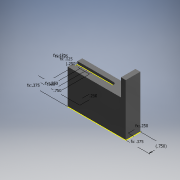
# Autodesk Inventor part: Spring block
Saved by Autodesk Inventor 2019 (Build 230136000, 136)
## iProperties
Part Number: Spring block
Material: Generic
Document SubType Name: Modeling
Designer: Delta
Appearance: Default
Author: Delta
Autodesk Inventor part; units mm, degrees
ref_plane "YZ Plane" through (0, 0, 0) normal (1, 0, 0) x (0, 1, 0)
ref_plane "XZ Plane" through (0, 0, 0) normal (0, 1, 0) x (-1, 0, 0)
ref_plane "XY Plane" through (0, 0, 0) normal (0, 0, 1) x (1, 0, 0)
sketch "Sketch1" plane through (0, 0, 0) normal (0, 0, 1) x (1, 0, 0)
  line L0 (0, 0) -> (76.2, 0)
  line L1 (76.2, 0) -> (76.2, 68.2498)
  line L2 (76.2, 68.2498) -> (0, 68.2498)
  line L3 (0, 68.2498) -> (0, 0)
  line L4 (0, 68.2498) -> (69.85, 68.2498)
  line L5 (69.85, 68.2498) -> (69.85, 45.3898)
  line L6 (69.85, 45.3898) -> (0, 45.3898)
  line L7 (0, 45.3898) -> (0, 68.2498)
  dimension "d0" = 76.2
  dimension "d1" = 68.2498
  dimension "d2" = 69.85
  dimension "d3" = 22.86
  constraints: 16 end point, 4 parallel, 2 horizontal, 2 perpendicular
  measures "d0" distance of L2.end L1.end
  measures "d1" distance of L1.end L0.end
  measures "d2" distance of L5.end L6.end
  measures "d3" distance of L4.end L5.end
extrude "Extrusion1" add sketch "Sketch1" along normal blind 19.05 contours L3 L6 L5 L2 L1 L0
sketch "Sketch2" plane through (0, 45.3898, 0) normal (0, 1, 0) x (1, 0, 0)
  line L0 (0, 0) -> (0, -19.05) projected
  line L1 (0, -6.35) -> (47.625, -6.35)
  line L2 (47.625, -6.35) -> (47.625, -12.7)
  line L3 (47.625, -12.7) -> (0, -12.7)
  line L4 (0, -12.7) -> (0, -6.35)
  line L5 (0, 0) -> (69.85, 0) projected
  circle A0 centre (47.625, -9.525) radius 3.175
  dimension "d6" = 47.625
  dimension "d7" = 6.35
  dimension "d8" = 6.35
  constraints: 8 end point, 2 parallel, 1 horizontal, 1 midpoint, 1 perpendicular, 1 point on line, 1 vertical alignment, 2 other
  measures "d6" distance of L2.end L3.end
  measures "d7" distance between parallel lines of L3 L1
  measures "d8" distance between parallel lines of L5 L1
extrude "Extrusion2" cut sketch "Sketch2" against normal blind 3.7084
sketch "Sketch3" plane through (0, 41.6814, 0) normal (0, 1, 0) x (1, 0, 0)
  line L0 (47.625, -12.7) -> (0, -12.7) projected
  line L1 (0, -6.35) -> (47.625, -6.35) projected
  line L2 (0, -12.7) -> (0, -6.35) projected
  point P0 (0, 0)
  point P1 (6.35, -9.525)
  point P2 (12.7, -9.525)
  point P3 (19.05, -9.525)
  dimension "d11" = 6.35
  dimension "d12" = 3.175
  dimension "d13" = 3.175
  dimension "d14" = 3.175
  dimension "d15" = 6.35
  dimension "d16" = 12.7
  dimension "d17" = 19.05
  measures "d11" distance between parallel lines of L0 L1
  measures "d12" distance from line of L0 point (6.35, -9.525)
  measures "d13" distance from line of point (12.7, -9.525) L0
  measures "d14" distance from line of L0 point (19.05, -9.525)
  measures "d15" distance from line of point (6.35, -9.525) L2
  measures "d16" distance from line of L2 point (12.7, -9.525)
  measures "d17" distance from line of point (19.05, -9.525) L2
sketch "Sketch4" plane through (0, 0, 0) normal (0, -1, 0) x (1, 0, 0)
  line L0 (0, 0) -> (76.2, 0) projected
  line L1 (0, 19.05) -> (76.2, 19.05) projected
  line L2 (0, 0) -> (0, 19.05) projected
  line L3 (76.2, 0) -> (76.2, 19.05) projected
  point P0 (6.35, 9.525)
  point P1 (69.85, 9.525)
  dimension "d18" = 19.05
  dimension "d19" = 9.525
  dimension "d20" = 9.525
  dimension "d21" = 6.35
  dimension "d22" = 6.35
  measures "d18" distance between parallel lines of L0 L1
  measures "d19" distance from line of L1 point (69.85, 9.525)
  measures "d20" distance from line of L1 point (6.35, 9.525)
  measures "d21" distance from line of point (6.35, 9.525) L2
  measures "d22" distance from line of L3 point (69.85, 9.525)
equation "\"d8\" = d7"
equation "\"d12\" = 0.5 * d11"
equation "\"d13\" = d12"
equation "\"d14\" = d13"
equation "\"d15\" = d11"
equation "\"d19\" = 0.5 * d18"
equation "\"d20\" = d19"
equation "\"d22\" = d21"
body "Solid1"
